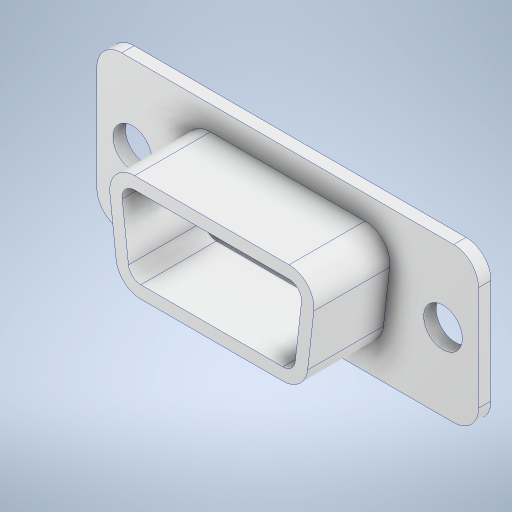
# Autodesk Inventor part: Dsub_9pin_female
Saved by Autodesk Inventor 2023 (Build 270158000, 158)
## iProperties
Created: 2023-06-03
Part Number: Dsub_9pin_female
Material: Aluminum 6061
Document SubType Name: Modeling
Designer: 310611102
Density: 2.7 g/cm^3
Appearance: Aluminum - Flat
Mass: 1.6702 g
Surface Area: 13.3943 cm^2
Volume: 0.618591 cm^3
Author: 310611102
Autodesk Inventor part; units mm, degrees
ref_plane "YZ Plane" through (0, 0, 0) normal (1, 0, 0) x (0, 1, 0)
ref_plane "XZ Plane" through (0, 0, 0) normal (0, 1, 0) x (-1, 0, 0)
ref_plane "XY Plane" through (0, 0, 0) normal (0, 0, 1) x (1, 0, 0)
sketch "Sketch1" plane through (0, 0, 0) normal (0, 0, 1) x (1, 0, 0)
  line L0 (-13.35, 6.2) -> (13.35, 6.2)
  line L1 (15.35, 4.2) -> (15.35, -4.2)
  line L2 (13.35, -6.2) -> (-13.35, -6.2)
  line L3 (-15.35, -4.2) -> (-15.35, 4.2)
  line L4 (-15.35, 6.2) -> (15.35, -6.2) construction
  line L5 (15.35, 6.2) -> (-15.35, -6.2) construction
  arc A0 (-13.35, 6.2) -> (-15.35, 4.2) centre (-13.35, 4.2) ccw
  arc A1 (15.35, 4.2) -> (13.35, 6.2) centre (13.35, 4.2) ccw
  arc A2 (13.35, -6.2) -> (15.35, -4.2) centre (13.35, -4.2) ccw
  arc A3 (-15.35, -4.2) -> (-13.35, -6.2) centre (-13.35, -4.2) ccw
  point P0 (0, 0)
  dimension "d0" = 12.4
  dimension "d1" = 30.7
  dimension "d2" = 2
  constraints: 12 end point, 8 point on circle, 8 point on line, 8 tangent, 4 centre point, 3 equal radius, 2 midpoint, 2 parallel, 1 horizontal, 1 perpendicular
  measures "d0" distance of L5.start L4.end
  measures "d1" distance of L4.start L5.start
  measures "d2" radius of A0
extrude "Extrusion1" add sketch "Sketch1" along normal blind 1
sketch "Sketch2" plane through (0, 0, 1) normal (0, 0, 1) x (1, 0, 0)
  circle A0 centre (-12.495, 0) radius 1.55
  circle A1 centre (12.495, 0) radius 1.55
  line L0 (0, 0) -> (0, 2.0374)
  dimension "d5" = 3.1
  dimension "d6" = 24.99
  constraints: 2 centre point, 2 end point, 1 equal radius, 1 horizontal alignment, 1 symmetric about line, 1 vertical
  measures "d5" diameter of A0
  measures "d6" distance of A1.centre A0.centre
extrude "Extrusion2" cut sketch "Sketch2" against normal through all
sketch "Sketch3" plane through (0, 0, 1) normal (0, 0, 1) x (1, 0, 0)
  line L0 (6.2132, 4.2657) -> (-6.2132, 4.2657)
  line L1 (-8.2003, 2.0385) -> (-7.7028, -2.3115)
  line L2 (-5.7157, -4.0843) -> (5.7157, -4.0843)
  line L3 (7.7028, -2.3115) -> (8.2003, 2.0385)
  line L4 (0, 0) -> (0, 9.8528)
  arc A0 (-6.2132, 4.2657) -> (-8.2003, 2.0385) centre (-6.2132, 2.2657) ccw
  arc A1 (8.2003, 2.0385) -> (6.2132, 4.2657) centre (6.2132, 2.2657) ccw
  arc A2 (5.7157, -4.0843) -> (7.7028, -2.3115) centre (5.7157, -2.0843) ccw
  arc A3 (-7.7028, -2.3115) -> (-5.7157, -4.0843) centre (-5.7157, -2.0843) ccw
  line L5 (6.2132, 2.2657) -> (-5.7157, -2.0843)
  line L6 (-6.2132, 2.2657) -> (5.7157, -2.0843)
  line L7 (-6.2132, 3.2657) -> (6.2132, 3.2657)
  arc A4 (7.2067, 2.1521) -> (6.2132, 3.2657) centre (6.2132, 2.2657) ccw
  line L8 (7.2067, 2.1521) -> (6.7092, -2.1979)
  arc A5 (5.7157, -3.0843) -> (6.7092, -2.1979) centre (5.7157, -2.0843) ccw
  line L9 (5.7157, -3.0843) -> (-5.7157, -3.0843)
  arc A6 (-6.7092, -2.1979) -> (-5.7157, -3.0843) centre (-5.7157, -2.0843) ccw
  line L10 (-6.7092, -2.1979) -> (-7.2067, 2.1521)
  arc A7 (-6.2132, 3.2657) -> (-7.2067, 2.1521) centre (-6.2132, 2.2657) ccw
  point P0 (8.455, 4.2657)
  point P1 (-8.455, 4.2657)
  point P2 (-7.5, -4.0843)
  point P3 (7.5, -4.0843)
  dimension "d9" = 8.35
  dimension "d10" = 16.91
  dimension "d11" = 15
  dimension "d12" = 2
  dimension "d15" = 1
  constraints: 22 end point, 16 point on circle, 10 point on line, 8 centre point, 8 tangent, 3 equal radius, 2 parallel, 1 coincident, 1 horizontal, 1 vertical, 8 other
  measures "d9" distance between parallel lines of L2 L0
  measures "d10" distance of point (-8.455, 4.266) point (8.455, 4.266)
  measures "d11" distance of point (-7.5, -4.084) point (7.5, -4.084)
  measures "d12" radius of A0
  measures "d15" distance between parallel lines of L0 L7
extrude "Extrusion3" add sketch "Sketch3" along normal blind 6.1
body "Solid1"
